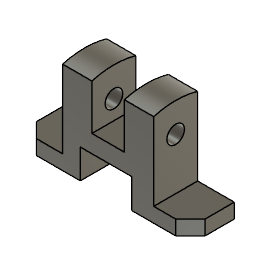
ISO 3 (Autodesk Fusion 360 design; units mm, degrees)
part number: 2026-02-06-09-43-23-762
Autodesk Fusion 360 part; units mm, degrees
sketch "Sketch1" plane through (0, 0, 0) normal (0, 1, 0) x (1, 0, 0)
  line L0 (-20, -5) -> (-20, 5)
  line L1 (-20, 5) -> (20, 5)
  line L2 (20, 5) -> (20, -15)
  line L3 (20, -15) -> (55, -15)
  line L4 (55, -15) -> (55, 5)
  line L5 (55, 5) -> (85, 5)
  line L6 (85, 5) -> (95, 5)
  line L7 (95, 5) -> (95, -5)
  line L8 (95, -5) -> (70, -5)
  line L9 (70, -5) -> (70, -60)
  line L10 (70, -60) -> (50, -60)
  line L11 (50, -60) -> (50, -27)
  line L12 (50, -27) -> (27.9096, -27)
  line L13 (27.9096, -27) -> (27.9096, -60)
  line L14 (27.9096, -60) -> (7.9096, -60)
  line L15 (7.9096, -60) -> (7.9096, -5)
  line L16 (7.9096, -5) -> (-20, -5)
  dimension "d2" = 20
  constraint vertical L0
  constraint perpendicular L0 L1
  constraint perpendicular L1 L2
  constraint perpendicular L0 L3
  constraint perpendicular L3 L4
  constraint perpendicular L4 L5
  constraint perpendicular L4 L6
  constraint perpendicular L6 L7
  constraint perpendicular L7 L8
  constraint perpendicular L8 L9
  constraint perpendicular L9 L10
  constraint perpendicular L3 L11
  constraint perpendicular L11 L12
  constraint perpendicular L12 L13
  constraint perpendicular L13 L14
  constraint perpendicular L14 L15
  constraint perpendicular L0 L16
  measures "d2" distance of L13.end L14.end
extrude "Extrude1" add sketch "Sketch1" along normal mid plane 30
chamfer "Chamfer1" distance 10 angle 45 2 edges at (-20, -15, 0) (95, -15, 0)
sketch "Sketch2" plane through (70, 0, 0) normal (1, 0, 0) x (0, 1, 0)
  line L0 (-15, 5) -> (15, 5)
  line L1 (15, 5) -> (15, 60)
  line L2 (15, 60) -> (-15, 60)
  line L3 (-15, 60) -> (-15, 5)
  point P0 (0, 40)
hole "Hole1" at (70, 0, 40) direction (-1, 0, 0) diameter 12 depth 65 tip angle 118
sketch "Sketch4" plane through (7.9096, 0, 0) normal (-1, 0, 0) x (0, -1, 0)
  circle A0 centre (0, 40) radius 6
  line L0 (15, 60) -> (-15, 60)
  line L1 (-15, 60) -> (-15, 5)
  line L2 (-15, 5) -> (15, 5)
  line L3 (15, 5) -> (15, 60)
  circle A1 centre (0, 5) radius 55
  constraint midpoint L2 A1.centre
extrude "Extrude2" cut sketch "Sketch4" against normal blind 12311 contours L0 L3 A1 | L0 L1 A1
